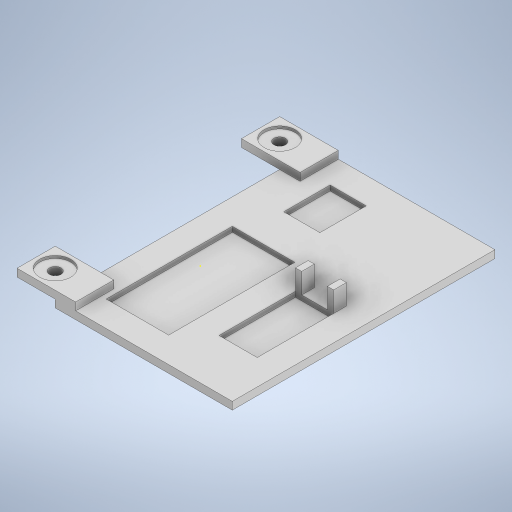
# Autodesk Inventor part: chrager_adapter
Saved by Autodesk Inventor 2024 (Build 280153000, 153)
## iProperties
Created: 2024-05-17
Part Number: chrager_adapter
Material: Generic
Document SubType Name: Modeling
Designer: inigo
Density: 1 g/cm^3
Appearance: Default
Author: inigo
Autodesk Inventor part; units mm, degrees
ref_plane "YZ Plane" through (0, 0, 0) normal (1, 0, 0) x (0, 1, 0)
ref_plane "XZ Plane" through (0, 0, 0) normal (0, 1, 0) x (-1, 0, 0)
ref_plane "XY Plane" through (0, 0, 0) normal (0, 0, 1) x (1, 0, 0)
sketch "Sketch1" plane through (0, 0, 0) normal (0, 1, 0) x (-1, 0, 0)
  line L0 (7.25, 29.75) -> (-17.25, 29.75)
  line L1 (-17.25, 29.75) -> (-17.25, -19.75)
  line L2 (-17.25, -19.75) -> (7.25, -19.75)
  line L3 (7.25, -19.75) -> (7.25, 29.75)
  line L4 (7.25, 29.75) -> (-17.25, -19.75) construction
  line L5 (-17.25, 29.75) -> (7.25, -19.75) construction
  line L6 (-27.25, 20) -> (-42.25, 20)
  line L7 (-42.25, 20) -> (-42.25, -10)
  line L8 (-42.25, -10) -> (-27.25, -10)
  line L9 (-27.25, -10) -> (-27.25, 20)
  line L10 (-27.25, 20) -> (-42.25, -10) construction
  line L11 (-42.25, 20) -> (-27.25, -10) construction
  line L12 (2.1, -34.75) -> (-12.1, -34.75)
  line L13 (-12.1, -34.75) -> (-12.1, -52.95)
  line L14 (-12.1, -52.95) -> (2.1, -52.95)
  line L15 (2.1, -52.95) -> (2.1, -34.75)
  line L16 (2.1, -34.75) -> (-12.1, -52.95) construction
  line L17 (-12.1, -34.75) -> (2.1, -52.95) construction
  line L18 (17.25, 39.75) -> (17.25, -51.55)
  line L19 (17.25, 24.75) -> (17.25, 39.75)
  line L20 (17.25, -36.55) -> (17.25, -51.55)
  line L21 (17.25, 39.75) -> (-52.25, 39.75)
  line L22 (-52.25, 39.75) -> (-52.25, -63.35)
  line L23 (-52.25, -63.35) -> (17.25, -63.35)
  line L24 (17.25, -63.35) -> (17.25, 39.75)
  point P0 (-34.75, 5)
  point P1 (-5, -43.85)
  point P2 (17.25, 0)
  dimension "d0" = 24.5
  dimension "d1" = 49.5
  dimension "d2" = 15
  dimension "d3" = 30
  dimension "d4" = 10
  dimension "d7" = 14.2
  dimension "d8" = 18.2
  dimension "d9" = 15
  dimension "d17" = 10
  dimension "d19" = 103.1
  dimension "d21" = 10
  dimension "d22" = 10
  constraints: 50 end point, 8 parallel, 4 horizontal, 4 midpoint, 4 perpendicular
  measures "d0" distance of L2.end L1.end
  measures "d1" distance of L1.end L0.end
  measures "d2" distance of L8.end L7.end
  measures "d3" distance of L7.end L6.end
  measures "d4" distance between parallel lines of L1 L9
  measures "d7" distance of L14.end L13.end
  measures "d8" distance of L13.end L12.end
  measures "d9" distance between parallel lines of L12 L2
  measures "d17" distance between parallel lines of L21 L0
  measures "d19" distance between parallel lines of L21 L23
  measures "d21" distance between parallel lines of L18 L3
  measures "d22" distance between parallel lines of L22 L7
extrude "Extrusion1" add sketch "Sketch1" along normal blind 3 contours L3 L2 L1 L0 | L9 L8 L7 L6 | L15 L14 L13 L12 | L18 L24 L23 L22 L21
sketch "Sketch2" plane through (0, 3, 0) normal (0, 1, 0) x (1, 0, 0)
  line L0 (-7.2398, -29.7311) -> (17.2602, -29.7311)
  line L1 (17.2602, -29.7311) -> (17.2602, 19.7689)
  line L2 (17.2602, 19.7689) -> (-7.2398, 19.7689)
  line L3 (-7.2398, 19.7689) -> (-7.2398, -29.7311)
  line L4 (-7.2398, -29.7311) -> (17.2602, 19.7689) construction
  line L5 (17.2602, -29.7311) -> (-7.2398, 19.7689) construction
  line L6 (27.2602, -19.9811) -> (42.2602, -19.9811)
  line L7 (42.2602, -19.9811) -> (42.2602, 10.0189)
  line L8 (42.2602, 10.0189) -> (27.2602, 10.0189)
  line L9 (27.2602, 10.0189) -> (27.2602, -19.9811)
  line L10 (27.2602, -19.9811) -> (42.2602, 10.0189) construction
  line L11 (42.2602, -19.9811) -> (27.2602, 10.0189) construction
  line L12 (-2.0898, 34.7689) -> (12.1102, 34.7689)
  line L13 (12.1102, 34.7689) -> (12.1102, 52.9689)
  line L14 (12.1102, 52.9689) -> (-2.0898, 52.9689)
  line L15 (-2.0898, 52.9689) -> (-2.0898, 34.7689)
  line L16 (-2.0898, 34.7689) -> (12.1102, 52.9689) construction
  line L17 (12.1102, 34.7689) -> (-2.0898, 52.9689) construction
  line L18 (-17.2398, -39.7311) -> (-17.2398, 51.5689)
  line L19 (-17.2398, -39.7311) -> (-32.2398, -39.7311)
  line L20 (-32.2398, -39.7311) -> (-32.2398, -24.7311)
  line L21 (-32.2398, -24.7311) -> (-17.2398, -24.7311)
  line L22 (-17.2398, -24.7311) -> (-17.2398, -39.7311)
  line L23 (-17.2398, 51.5689) -> (-32.2398, 51.5689)
  line L24 (-32.2398, 51.5689) -> (-32.2398, 36.5689)
  line L25 (-32.2398, 36.5689) -> (-17.2398, 36.5689)
  line L26 (-17.2398, 36.5689) -> (-17.2398, 51.5689)
  line L27 (-17.2398, -39.7311) -> (52.2602, -39.7311)
  line L28 (52.2602, -39.7311) -> (52.2602, 63.3689)
  line L29 (52.2602, 63.3689) -> (-17.2398, 63.3689)
  line L30 (-17.2398, 63.3689) -> (-17.2398, -39.7311)
  point P0 (0, 0)
  point P1 (34.7602, -4.9811)
  point P2 (5.0102, 43.8689)
  point P3 (-17.2398, 0.0189)
  dimension "d25" = 24.5
  dimension "d26" = 49.5
  dimension "d27" = 15
  dimension "d28" = 30
  dimension "d29" = 10
  dimension "d30" = 14.2
  dimension "d31" = 18.2
  dimension "d32" = 15
  dimension "d33" = 15
  dimension "d34" = 15
  dimension "d35" = 15
  dimension "d36" = 15
  dimension "d37" = 10
  dimension "d38" = 11.8
  dimension "d39" = 103.1
  dimension "d40" = 10
  dimension "d41" = 10
  constraints: 62 end point, 12 parallel, 6 perpendicular, 4 midpoint
  measures "d25" distance of L3.start L4.end
  measures "d26" distance of L4.end L5.start
  measures "d27" distance of L9.start L8.start
  measures "d28" distance of L8.start L6.end
  measures "d29" distance between parallel lines of L1 L9
  measures "d30" distance of L15.start L13.end
  measures "d31" distance of L13.end L13.start
  measures "d32" distance between parallel lines of L12 L2
  measures "d33" distance of L21.start L22.start
  measures "d34" distance of L20.start L21.start
  measures "d35" distance of L26.start L24.end
  measures "d36" distance of L24.end L24.start
  measures "d37" distance between parallel lines of L27 L0
  measures "d38" distance between parallel lines of L29 L23
  measures "d39" distance between parallel lines of L27 L29
  measures "d40" distance between parallel lines of L18 L3
  measures "d41" distance between parallel lines of L28 L7
extrude "Extrusion2" cut sketch "Sketch2" against normal blind 2 contours L3 L2 L1 L0 | L9 L8 L7 L6 | L15 L14 L13 L12
sketch "Sketch3" plane through (0, 3, 0) normal (0, 1, 0) x (1, 0, 0)
  point P0 (0, 0)
sketch "Sketch4" plane through (0, 3, 0) normal (0, 1, 0) x (1, 0, 0)
  line L0 (29.7102, 15.7954) -> (39.8102, 15.7954)
  line L1 (39.8102, 15.7954) -> (39.8102, 4.2425)
  line L2 (39.8102, 4.2425) -> (29.7102, 4.2425)
  line L3 (29.7102, 4.2425) -> (29.7102, 15.7954)
  line L4 (27.2602, 10.0189) -> (42.2602, 10.0189) projected
  line L5 (29.7102, 15.7954) -> (39.8102, 4.2425) construction
  line L6 (39.8102, 15.7954) -> (29.7102, 4.2425) construction
  line L7 (27.2602, 10.0189) -> (29.7102, 10.0189)
  line L8 (29.7102, 10.0189) -> (29.7102, 15.0189)
  line L9 (29.7102, 15.0189) -> (27.2602, 15.0189)
  line L10 (27.2602, 15.0189) -> (27.2602, 10.0189)
  line L11 (42.2602, 10.0189) -> (39.8102, 10.0189)
  line L12 (39.8102, 10.0189) -> (39.8102, 15.0189)
  line L13 (39.8102, 15.0189) -> (42.2602, 15.0189)
  line L14 (42.2602, 15.0189) -> (42.2602, 10.0189)
  point P0 (0, 0)
  point P1 (34.7602, 10.0189)
  point P2 (39.8102, 10.0189)
  point P3 (29.7102, 10.0189)
  dimension "d44" = 10.1
  dimension "d45" = 5
  dimension "d46" = 5
  constraints: 28 end point, 6 parallel, 3 horizontal, 3 midpoint, 3 perpendicular, 2 point on line
  measures "d44" distance of L1.end L2.end
  measures "d45" distance of L8.end L7.end
  measures "d46" distance of L11.end L12.end
extrude "Extrusion3" add sketch "Sketch4" along normal blind 8 contours L3 L4 L10 L9 | L13 L14 L4 L1
sketch "Sketch7" plane through (0, 3, 0) normal (0, 1, 0) x (1, 0, 0)
  line L0 (-17.25, -39.75) -> (-32.25, -39.75)
  line L1 (-32.25, -39.75) -> (-32.25, -24.75)
  line L2 (-32.25, -24.75) -> (-17.25, -24.75)
  line L3 (-17.25, -24.75) -> (-17.25, -39.75)
  line L4 (52.25, 63.35) -> (-17.25, 63.35) projected
  line L5 (-17.25, 63.35) -> (-32.25, 63.35)
  line L6 (-32.25, 63.35) -> (-32.25, 48.35)
  line L7 (-32.25, 48.35) -> (-17.25, 48.35)
  line L8 (-17.25, 48.35) -> (-17.25, 63.35)
  line L9 (-17.25, -39.75) -> (-9.25, -39.75)
  line L10 (-9.25, -39.75) -> (-9.25, -24.75)
  line L11 (-9.25, -24.75) -> (-17.25, -24.75)
  line L12 (-17.25, -24.75) -> (-17.25, -39.75)
  line L13 (-17.25, 48.35) -> (-9.25, 48.35)
  line L14 (-9.25, 48.35) -> (-9.25, 63.35)
  line L15 (-9.25, 63.35) -> (-17.25, 63.35)
  line L16 (-17.25, 63.35) -> (-17.25, 48.35)
  point P0 (0, 0)
  dimension "d52" = 15
  dimension "d53" = 15
  dimension "d54" = 15
  dimension "d55" = 15
  dimension "d56" = 8
  constraints: 32 end point, 8 parallel, 4 horizontal, 4 perpendicular, 2 point on line
  measures "d52" distance of L1.end L2.end
  measures "d53" distance of L0.end L1.end
  measures "d54" distance of L7.end L6.end
  measures "d55" distance of L6.end L5.end
  measures "d56" distance of L11.end L10.end
extrude "Extrusion5" add sketch "Sketch7" along normal blind 3
sketch "Sketch8" plane through (0, 6, 0) normal (0, 1, 0) x (1, 0, 0)
  line L0 (-32.25, -24.75) -> (-32.25, -39.75) projected
  line L1 (-9.25, -24.75) -> (-32.25, -24.75) projected
  line L2 (-17.25, 63.35) -> (-17.25, -39.75) projected
  line L3 (-17.25, -24.75) -> (-32.25, -24.75)
  circle A0 centre (-24.75, -32.25) radius 2.25
  circle A1 centre (-24.75, 55.85) radius 2.25
  point P0 (0, 0)
  dimension "d59" = 4.5
  dimension "d60" = 4.5
  constraints: 2 centre point, 2 end point, 2 point on line, 1 perpendicular
  measures "d59" diameter of A0
  measures "d60" diameter of A1
extrude "Extrusion6" cut sketch "Sketch8" against normal blind 3
sketch "Sketch9" plane through (0, 6, 0) normal (0, 1, 0) x (1, 0, 0)
  circle A0 centre (-24.75, -32.25) radius 2.25 projected
  circle A1 centre (-24.75, -32.25) radius 6.1
  circle A2 centre (-24.75, 55.85) radius 2.25 projected
  circle A3 centre (-24.75, 55.85) radius 6.1
  point P0 (0, 0)
  dimension "d63" = 12.2
  dimension "d64" = 12.2
  constraints: 2 centre point, 2 coincident
  measures "d63" diameter of A1
  measures "d64" diameter of A3
extrude "Extrusion7" cut sketch "Sketch9" against normal blind 1 contours A0 | A1 | A3
sketch "Sketch10" plane through (0, 3, 0) normal (0, -1, 0) x (1, 0, 0)
  circle A0 centre (-24.75, 32.25) radius 2.25 projected
  circle A1 centre (-24.75, 32.25) radius 6.1
  circle A2 centre (-24.75, -55.85) radius 2.25 projected
  circle A3 centre (-24.75, -55.85) radius 6.1
  point P0 (0, 0)
  dimension "d67" = 12.2
  dimension "d68" = 12.2
  constraints: 2 centre point, 2 coincident
  measures "d67" diameter of A1
  measures "d68" diameter of A3
extrude "Extrusion8" add sketch "Sketch10" along normal blind 1
body "Solid1"
